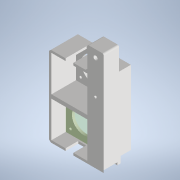
# Autodesk Inventor part: 30_XYTable_Aliexpress_motormount
Saved by Autodesk Inventor 2022 (Build 260153000, 153)
## iProperties
Created: 2021-11-19
Part Number: 30_XYTable_Aliexpress_motormount
Material: Generic
Document SubType Name: Modeling
Designer: diederichbenedict
Density: 1 g/cm^3
Appearance: Default
Author: diederichbenedict
Autodesk Inventor part; units mm, degrees
sketch "Sketch1" plane through (0, 0, 0) normal (0, 0, 1) x (1, 0, 0)
  line L0 (0, 0) -> (-19.7, 0)
  line L1 (-19.7, 0) -> (-19.7, 180)
  line L2 (-19.7, 180) -> (0, 180)
  line L3 (0, 180) -> (0, 38)
  line L4 (0, 38) -> (-19.7, 38)
  dimension "d0" = 19.7
  dimension "d1" = 180
  dimension "d53" = 142
  constraints: 10 end point, 2 parallel, 2 perpendicular, 1 horizontal, 1 point on line
  measures "d0" distance of L1.end L2.end
  measures "d1" distance of L0.end L1.end
  measures "d53" distance between parallel lines of L4 L2
extrude "Extrusion1" add sketch "Sketch1" along normal blind 18
fillet "Fillet1" radius 2 2 edges at (0, 180, 9) (-19.7, 180, 9)
sketch "Sketch2" plane through (0, 0, 0) normal (0, 0, -1) x (-1, 0, 0)
  line L0 (19.7, 178) -> (19.7, 38) projected
  arc A0 (19.7, 178) -> (17.7, 180) centre (17.7, 178) ccw projected
  line L1 (2, 180) -> (17.7, 180) projected
  arc A1 (2, 180) -> (0, 178) centre (2, 178) ccw projected
  line L2 (0, 38) -> (0, 178) projected
  line L3 (-8.568, 22) -> (7.7, 22) construction
  line L4 (-8.568, 12) -> (7.7, 12)
  line L5 (7.7, 32) -> (-8.568, 32)
  arc A2 (-8.568, 32) -> (-8.568, 12) centre (-8.568, 22) ccw
  arc A3 (7.7, 12) -> (7.7, 32) centre (7.7, 22) ccw
  line L6 (19.7, 38) -> (0, 38) projected
  point P0 (0, 0)
  point P1 (-0.434, 22)
  dimension "d5" = 20
  dimension "d6" = 12
  constraints: 8 end point, 4 point on circle, 4 tangent, 2 centre point, 1 horizontal, 1 midpoint, 1 parallel
  measures "d5" diameter of A3
  measures "d6" distance from line of L3.end L0
extrude "Extrusion2" cut sketch "Sketch2" against normal blind 9 contours A2 L5 A3 L4
sketch "Sketch4" plane through (0, 0, 0) normal (0, 0, -1) x (-1, 0, 0)
  line L0 (0, 38) -> (0, 178) projected
  line L1 (19.7, 178) -> (19.7, 38) projected
  arc A0 (19.7, 178) -> (17.7, 180) centre (17.7, 178) ccw projected
  line L2 (2, 180) -> (17.7, 180) projected
  arc A1 (2, 180) -> (0, 178) centre (2, 178) ccw projected
  circle A2 centre (9.7, 52) radius 1.5
  circle A3 centre (9.7, 131) radius 1.5
  line L3 (19.7, 38) -> (0, 38) projected
  point P0 (0, 0)
  dimension "d14" = 3
  dimension "d15" = 3
  dimension "d16" = 10
  dimension "d17" = 10
  dimension "d18" = 49
  dimension "d19" = 79
  constraints: 2 centre point
  measures "d14" diameter of A2
  measures "d15" diameter of A3
  measures "d16" distance from line of A3.centre L1
  measures "d17" distance from line of L1 A2.centre
  measures "d18" distance from line of A3.centre L2
  measures "d19" distance of A2.centre A3.centre
extrude "Extrusion4" cut sketch "Sketch4" against normal blind 110 contours A2 | A3
ref_plane "Work Plane1" through (-61.2, 108.5, -24) normal (0, 0, -1) x (0, 1, 0)
ref_plane "Work Plane3" through (-61.2, 108.5, -11) normal (0, 0, -1) x (0, 1, 0)
sketch "Sketch5" plane through (0, 0, 18) normal (0, 0, 1) x (1, 0, 0)
  circle A0 centre (-9.7, 52) radius 1.5
  circle A1 centre (-9.7, 131) radius 1.5
  line L0 (0, 38) -> (0, 178)
  arc A2 (0, 178) -> (-2, 180) centre (-2, 178) ccw
  line L1 (-2, 180) -> (-17.7, 180)
  arc A3 (-17.7, 180) -> (-19.7, 178) centre (-17.7, 178) ccw
  line L2 (-19.7, 178) -> (-19.7, 38)
  line L3 (-23.7294, 108) -> (-57.6706, 108)
  line L4 (-57.4929, 102.5) -> (-23.9071, 102.5)
  line L5 (-57.6706, 103) -> (-23.7294, 103)
  line L6 (-19.7, 178) -> (-19.7, 38)
  line L7 (-19.7, 108) -> (-61.7, 108)
  line L8 (-61.7, 108) -> (-61.7, 103)
  line L9 (-61.7, 103) -> (-19.7, 103)
  line L10 (-19.7, 103) -> (-19.7, 108)
  line L11 (-61.7, 112.0294) -> (-61.7, 145.9706)
  line L12 (-57.6706, 150) -> (-23.7294, 150)
  line L13 (-23.7294, 61) -> (-57.6706, 61)
  line L14 (0, 38) -> (0, 178)
  line L15 (-19.7, 150) -> (0, 150)
  line L16 (0, 150) -> (0, 61)
  line L17 (0, 61) -> (-19.7, 61)
  line L18 (-19.7, 61) -> (-19.7, 150)
  line L19 (-19.7, 38) -> (0, 38)
  point P0 (0, 0)
  point P1 (0, 110)
  point P2 (-19.7, 2)
  point P3 (0, 32)
  point P4 (-19.7, 103)
  point P5 (-19.7, 103)
extrude "Extrusion5" add sketch "Sketch5" against normal up to surface (29 mm away) contours L17 L2 L15 L0 | L9 L5 L8 L7 L3 L2
sketch "Sketch6" plane through (-19.7, 103, -11) normal (0, 0, -1) x (-1, 0, 0)
  circle A0 centre (-10, 28) radius 1.5 projected
  line L0 (0, -42) -> (-19.7, -42) projected
  line L1 (0, 0) -> (0, -42) projected
  line L2 (42, 0) -> (0, 0) projected
  line L3 (42, 5) -> (42, 0) projected
  line L4 (0, 5) -> (42, 5) projected
  line L5 (0, 47) -> (0, 5) projected
  line L6 (-19.7, 47) -> (0, 47) projected
  line L7 (-19.7, -42) -> (-19.7, 47) projected
  line L8 (0, 5) -> (42, 5) projected
  line L9 (0, 75) -> (0, 47) projected
  line L10 (42, 5) -> (0, 5)
  line L11 (0, 5) -> (0, 47)
  line L12 (0, 47) -> (42, 47)
  line L13 (42, 47) -> (42, 5)
  circle A1 centre (36.5, 10.5) radius 1.5 projected
  circle A2 centre (5.5, 10.5) radius 1.5 projected
  circle A3 centre (5.5, 41.5) radius 1.5 projected
  circle A4 centre (36.5, 41.5) radius 1.5 projected
  circle A5 centre (21, 26) radius 15 projected
  point P0 (-19.7, -103)
  constraints: 8 end point, 2 parallel, 1 horizontal, 1 perpendicular
extrude "Extrusion6" add sketch "Sketch6" along normal blind 3
ref_plane "Work Plane2" through (-40.7, 82, 1) normal (0, 0, -1) x (1, 0, 0)
sketch "Sketch7" plane through (-40.7, 82, 1) normal (0, 0, -1) x (1, 0, 0)
  line L0 (-21, -68) -> (40.7, -68) projected
  line L1 (40.7, -68) -> (40.7, 21) projected
  line L2 (40.7, 21) -> (21, 21) projected
  line L3 (21, 21) -> (21, -21) projected
  line L4 (21, -21) -> (-21, -21) projected
  line L5 (-21, -21) -> (-21, -68) projected
  circle A0 centre (31, -49) radius 1.5 projected
  circle A1 centre (0, -47) radius 15 projected
  circle A2 centre (-15.5, -62.5) radius 1.5 projected
  circle A3 centre (15.5, -62.5) radius 1.5 projected
  circle A4 centre (15.5, -31.5) radius 1.5 projected
  circle A5 centre (-15.5, -31.5) radius 1.5 projected
  line L6 (21, 21) -> (40.7, 21) projected
  line L7 (21, -21) -> (-21, -21) projected
  line L8 (21, 21) -> (-21, 21)
  line L9 (-21, 21) -> (-21, -21)
  line L10 (-21, -21) -> (21, -21)
  line L11 (21, -21) -> (21, 21)
  circle A6 centre (-15.5, 15.5) radius 1.5 projected
  circle A7 centre (-15.5, -15.5) radius 1.5 projected
  circle A8 centre (15.5, -15.5) radius 1.5 projected
  circle A9 centre (15.5, 15.5) radius 1.5 projected
  circle A10 centre (0, 0) radius 14 projected
  point P0 (40.7, 82)
  point P1 (34.7, 21)
  constraints: 8 end point, 2 parallel, 1 horizontal, 1 perpendicular
extrude "Extrusion7" add sketch "Sketch7" along normal blind 3 contours L9 L8 L3 L4
sketch "Sketch8" plane through (-61.7, 103, 18) normal (-1, 0, 0) x (0, 0, 1)
  line L0 (0, 0) -> (-17, 0) projected
  line L1 (0, 5) -> (0, 0) projected
  line L2 (0, 5) -> (-29, 5) projected
  line L3 (-29, 5) -> (-29, 47) projected
  line L4 (-29, 47) -> (-32, 47) projected
  line L5 (-32, 0) -> (-32, 47) projected
  line L6 (-20, 0) -> (-32, 0) projected
  line L7 (-20, -42) -> (-20, 0) projected
  line L8 (-17, -42) -> (-20, -42) projected
  line L9 (-17, -42) -> (-17, 0) projected
  line L10 (-32, 47) -> (-32, -42) projected
  line L11 (-32, 47) -> (0, 47)
  line L12 (0, 47) -> (0, 0)
  line L13 (0, 0) -> (-32, 0)
  line L14 (-32, 0) -> (-32, 47)
  line L15 (0, 0) -> (-20, 0)
  line L16 (-20, 0) -> (-20, -42)
  line L17 (-20, -42) -> (0, -42)
  line L18 (0, -42) -> (0, 0)
  point P0 (-18, -103)
  point P1 (-23, 7)
  constraints: 16 end point, 4 parallel, 2 horizontal, 2 perpendicular, 2 other
extrude "Extrusion8" add sketch "Sketch8" along normal blind 3
sketch "Sketch9" plane through (-19.7, 150, 0) normal (0, 1, 0) x (1, 0, 0)
  line L0 (19.7, 0) -> (0, 0) projected
  line L1 (19.7, 0) -> (19.7, 14) projected
  line L2 (19.7, 14) -> (-45, 14) projected
  line L3 (-45, -18) -> (-45, 14) projected
  line L4 (-42, -18) -> (-45, -18) projected
  line L5 (-42, -18) -> (-42, 11) projected
  line L6 (-42, 11) -> (0, 11) projected
  line L7 (0, 0) -> (0, 11) projected
  line L8 (-42, -18) -> (0, -18) projected
  line L9 (-42, 11) -> (0, 11) projected
  line L10 (-42, -18) -> (0, -18)
  line L11 (0, -18) -> (0, 11)
  line L12 (0, 11) -> (-42, 11)
  line L13 (-42, 11) -> (-42, -18)
  constraints: 8 end point, 2 parallel, 1 horizontal, 1 perpendicular
extrude "Extrusion9" add sketch "Sketch9" along normal blind 3
sketch "Sketch10" plane through (-19.7, 61, 0) normal (0, -1, 0) x (1, 0, 0)
  line L0 (0, 0) -> (19.7, 0) projected
  line L1 (0, 1) -> (0, 0) projected
  line L2 (0, 1) -> (-42, 1) projected
  line L3 (-42, 1) -> (-42, 18) projected
  line L4 (-42, 18) -> (-45, 18) projected
  line L5 (-45, -2) -> (-45, 18) projected
  line L6 (0, -2) -> (-45, -2) projected
  line L7 (0, -2) -> (0, -14) projected
  line L8 (19.7, -14) -> (0, -14) projected
  line L9 (-42, 1) -> (0, 1) projected
  line L10 (0, -11) -> (0, 18) projected
  line L11 (-42, 1) -> (0, 1)
  line L12 (0, 1) -> (0, 18)
  line L13 (0, 18) -> (-42, 18)
  line L14 (-42, 18) -> (-42, 1)
  line L15 (19.7, 0) -> (19.7, -14) projected
  point P0 (19.7, 0)
  constraints: 8 end point, 2 parallel, 1 horizontal, 1 perpendicular
extrude "Extrusion10" add sketch "Sketch10" along normal blind 3
sketch "Sketch11" plane through (0, 0, 18) normal (0, 0, 1) x (1, 0, 0)
  line L0 (-61.7, 61) -> (-61.7, 103) projected
  line L1 (-61.7, 103) -> (-19.7, 103) projected
  line L2 (-19.7, 103) -> (-19.7, 61) projected
  line L3 (-19.7, 61) -> (-61.7, 61) projected
  line L4 (-19.7, 150) -> (-19.7, 108) projected
  line L5 (-19.7, 108) -> (-61.7, 108) projected
  line L6 (-61.7, 108) -> (-61.7, 150) projected
  line L7 (-61.7, 150) -> (-19.7, 150) projected
  circle A0 centre (-9.7, 52) radius 1.5 projected
  circle A1 centre (-9.7, 131) radius 1.5 projected
  line L8 (-64.7, 153) -> (-64.7, 58) projected
  line L9 (-19.7, 58) -> (-64.7, 58) projected
  line L10 (-19.7, 58) -> (-19.7, 38) projected
  line L11 (0, 38) -> (0, 178) projected
  arc A2 (0, 178) -> (-2, 180) centre (-2, 178) ccw projected
  line L12 (-2, 180) -> (-17.7, 180) projected
  arc A3 (-17.7, 180) -> (-19.7, 178) centre (-17.7, 178) ccw projected
  line L13 (-19.7, 178) -> (-19.7, 153) projected
  line L14 (-64.7, 153) -> (-19.7, 153) projected
  line L15 (-61.95, 103.25) -> (-61.95, 60.75)
  line L16 (-61.95, 60.75) -> (-19.45, 60.75)
  line L17 (-19.45, 60.75) -> (-19.45, 103.25)
  line L18 (-19.45, 103.25) -> (-61.95, 103.25)
  line L19 (-61.95, 150.25) -> (-61.95, 107.75)
  line L20 (-61.95, 107.75) -> (-19.45, 107.75)
  line L21 (-19.45, 107.75) -> (-19.45, 150.25)
  line L22 (-19.45, 150.25) -> (-61.95, 150.25)
  line L23 (-19.7, 38) -> (0, 38) projected
  point P0 (0, 0)
  dimension "d35" = 0.25
  dimension "d36" = 0.25
  constraints: 16 end point, 6 other
  measures "d35" distance between parallel lines of L0 L15
  measures "d36" distance between parallel lines of L6 L19
extrude "Extrusion11" cut sketch "Sketch11" against normal up to surface (17 mm away) contours L0 L1 L2 L3 | L4 L5 L6 L7 | L18 L17 L16 L15 | L22 L21 L20 L19
sketch "Sketch12" plane through (0, 0, 18) normal (0, 0, 1) x (1, 0, 0)
  line L0 (-61.95, 107.75) -> (-61.95, 150.25) projected
  line L1 (-61.95, 150.25) -> (-19.45, 150.25) projected
  line L2 (-19.45, 150.25) -> (-19.45, 107.75) projected
  line L3 (-19.45, 107.75) -> (-61.95, 107.75) projected
  line L4 (-61.95, 103.25) -> (-19.45, 103.25) projected
  line L5 (-19.45, 103.25) -> (-19.45, 60.75) projected
  line L6 (-19.45, 60.75) -> (-61.95, 60.75) projected
  line L7 (-61.95, 60.75) -> (-61.95, 103.25) projected
  circle A0 centre (-9.7, 52) radius 1.5 projected
  circle A1 centre (-9.7, 131) radius 1.5 projected
  line L8 (-64.7, 153) -> (-64.7, 58) projected
  line L9 (-19.7, 58) -> (-64.7, 58) projected
  line L10 (-19.7, 58) -> (-19.7, 38) projected
  line L11 (0, 38) -> (0, 178) projected
  arc A2 (0, 178) -> (-2, 180) centre (-2, 178) ccw projected
  line L12 (-2, 180) -> (-17.7, 180) projected
  arc A3 (-17.7, 180) -> (-19.7, 178) centre (-17.7, 178) ccw projected
  line L13 (-19.7, 178) -> (-19.7, 153) projected
  line L14 (-64.7, 153) -> (-19.7, 153) projected
  line L15 (-19.7, 38) -> (0, 38) projected
  point P0 (0, 0)
ref_plane "Work Plane4" through (-61.2, 108.5, -11) normal (0, 0, -1) x (0, 1, 0)
extrude "Extrusion12" cut sketch "Sketch12" against normal up to surface (29 mm away) contours L0 L1 L2 L3
chamfer "Chamfer1" distance 2 angle 45 6 edges at (-64.7, 58, 8) (-64.7, 153, 2) (-64.7, 103, -8) (-19.7, 58, 9) (-19.7, 58, -8) (-19.7, 153, 9)
sketch "Sketch13" plane through (-19.7, 103, -14) normal (0, 0, -1) x (-1, 0, 0)
  circle A0 centre (-10, 28) radius 1.5 projected
  circle A1 centre (-10, -51) radius 1.5 projected
  point P0 (-19.7, -103)
hole "Hole1" at (-9.7, 52, -14) at (-9.7, 131, -14) direction (0, 0, 1) diameter 2.5 end through all counterbore diameter 5 counterbore depth 20
sketch "Sketch14" plane through (-19.7, 103, -14) normal (0, 0, -1) x (-1, 0, 0)
  circle A0 centre (-10, 28) radius 2.5 projected
  circle A1 centre (36.5, 10.5) radius 1.5 projected
  circle A2 centre (5.5, 10.5) radius 1.5 projected
  circle A3 centre (5.5, 41.5) radius 1.5 projected
  circle A4 centre (36.5, 41.5) radius 1.5 projected
  circle A5 centre (21, 26) radius 15 projected
  line L0 (0, -43) -> (-2, -45) projected
  line L1 (0, 0) -> (0, -43) projected
  line L2 (0, 0) -> (43, 0) projected
  line L3 (45, 2) -> (43, 0) projected
  line L4 (45, 2) -> (45, 48) projected
  line L5 (43, 50) -> (45, 48) projected
  line L6 (-19.7, 50) -> (43, 50) projected
  line L7 (-19.7, -45) -> (-19.7, 50) projected
  line L8 (-2, -45) -> (-19.7, -45) projected
  circle A6 centre (21, -21) radius 3.5 projected
  line L9 (-32.7587, -50.6684) -> (7.6884, -72.8519)
  line L10 (7.6884, -72.8519) -> (27.6493, -33.2508)
  circle A7 centre (21, -21) radius 14 projected
  line L11 (27.6013, -33.346) -> (5.5, -11.6661)
  line L12 (5.5, -11.6661) -> (-32.7587, -50.6684)
  point P0 (-19.7, -103)
  point P1 (18.9527, -18.1612)
  constraints: 8 end point, 1 perpendicular, 1 point on line, 4 other
extrude "Extrusion13" cut sketch "Sketch14" against normal up to surface (12 mm away) contours L1 L12 L11 A7 L10 L9 L7 L8 L0 | L0 L8 L7 L12 L1 | L11 A7 | A6 picked at (13.3334, -27.485)
sketch "Sketch15" plane through (0, 0, -14) normal (0, 0, -1) x (-1, 0, 0)
  circle A0 centre (9.7, 52) radius 2.5 projected
  circle A1 centre (9.5, 171.1) radius 2.5
  line L0 (2, 180) -> (17.7, 180) projected
  line L1 (0, 153) -> (0, 178) projected
  circle A2 centre (9.85, 121.1) radius 2.9049
  circle A3 centre (9.5, 61.1) radius 2.7549
  point P0 (0, 0)
  dimension "d54" = 5
  dimension "d55" = 8.9
  dimension "d70" = 9.5
  dimension "d71" = 50
  dimension "d72" = 60
  constraints: 3 centre point
  measures "d54" diameter of A1
  measures "d55" distance from line of A1.centre L0
  measures "d70" distance from line of A1.centre L1
  measures "d71" vertical distance of A2.centre A1.centre
  measures "d72" vertical distance of A3.centre A2.centre
sketch "Skizze16" plane through (0, 0, 18) normal (0, 0, 1) x (1, 0, 0)
  line L0 (-64.7, 151) -> (-62.7, 153) projected
  line L1 (-64.7, 151) -> (-64.7, 60) projected
  line L2 (-62.7, 58) -> (-64.7, 60) projected
  line L3 (-21.7, 58) -> (-62.7, 58) projected
  line L4 (-19.7, 56) -> (-21.7, 58) projected
  line L5 (-19.7, 56) -> (-19.7, 38) projected
  line L6 (-19.7, 38) -> (0, 38) projected
  line L7 (0, 38) -> (0, 178) projected
  arc A0 (0, 178) -> (-2, 180) centre (-2, 178) ccw projected
  line L8 (-2, 180) -> (-17.7, 180) projected
  arc A1 (-17.7, 180) -> (-19.7, 178) centre (-17.7, 178) ccw projected
  line L9 (-19.7, 178) -> (-19.7, 155) projected
  line L10 (-21.7, 153) -> (-19.7, 155) projected
  line L11 (-62.7, 153) -> (-21.7, 153) projected
  line L12 (-61.95, 107.75) -> (-61.95, 150.25) projected
  line L13 (-61.95, 150.25) -> (-19.45, 150.25) projected
  line L14 (-19.45, 150.25) -> (-19.45, 107.75) projected
  line L15 (-19.45, 107.75) -> (-61.95, 107.75) projected
  line L16 (-61.95, 103.25) -> (-19.45, 103.25) projected
  line L17 (-19.45, 103.25) -> (-19.45, 60.75) projected
  line L18 (-19.45, 60.75) -> (-61.95, 60.75) projected
  line L19 (-61.95, 60.75) -> (-61.95, 103.25) projected
  circle A2 centre (-9.7, 52) radius 1.5 projected
  circle A3 centre (-9.7, 131) radius 1.5 projected
  line L20 (-45.3346, 64) -> (-36.0654, 64)
  line L21 (-36.0654, 64) -> (-36.0654, 56)
  line L22 (-36.0654, 56) -> (-45.3346, 56)
  line L23 (-45.3346, 56) -> (-45.3346, 64)
  line L24 (-45.3346, 64) -> (-36.0654, 56) construction
  line L25 (-36.0654, 64) -> (-45.3346, 56) construction
  point P0 (0, 0)
  point P1 (-40.7, 60)
  constraints: 12 end point, 2 midpoint, 2 parallel, 1 horizontal, 1 perpendicular
extrude "Extrusion15" cut sketch "Skizze16" against normal blind 15 contours L23 L18 L21 L3 | L3 L21 L22 L23 | L23 L20 L21 L18
sketch "Skizze17" plane through (0, 0, 18) normal (0, 0, 1) x (1, 0, 0)
  line L0 (-36.0654, 60.75) -> (-36.0654, 58) projected
  line L1 (-21.7, 58) -> (-36.0654, 58) projected
  line L2 (-19.7, 56) -> (-21.7, 58) projected
  line L3 (-19.7, 56) -> (-19.7, 38) projected
  line L4 (-19.7, 38) -> (0, 38) projected
  line L5 (0, 38) -> (0, 178) projected
  arc A0 (0, 178) -> (-2, 180) centre (-2, 178) ccw projected
  line L6 (-2, 180) -> (-17.7, 180) projected
  arc A1 (-17.7, 180) -> (-19.7, 178) centre (-17.7, 178) ccw projected
  line L7 (-19.7, 178) -> (-19.7, 155) projected
  line L8 (-21.7, 153) -> (-19.7, 155) projected
  line L9 (-62.7, 153) -> (-21.7, 153) projected
  line L10 (-64.7, 151) -> (-62.7, 153) projected
  line L11 (-64.7, 151) -> (-64.7, 60) projected
  line L12 (-62.7, 58) -> (-64.7, 60) projected
  line L13 (-45.3346, 58) -> (-62.7, 58) projected
  line L14 (-45.3346, 58) -> (-45.3346, 60.75) projected
  line L15 (-45.3346, 60.75) -> (-61.95, 60.75) projected
  line L16 (-61.95, 60.75) -> (-61.95, 103.25) projected
  line L17 (-61.95, 103.25) -> (-19.45, 103.25) projected
  line L18 (-19.45, 103.25) -> (-19.45, 60.75) projected
  line L19 (-19.45, 60.75) -> (-36.0654, 60.75) projected
  line L20 (-61.95, 107.75) -> (-61.95, 150.25) projected
  line L21 (-61.95, 150.25) -> (-19.45, 150.25) projected
  line L22 (-19.45, 150.25) -> (-19.45, 107.75) projected
  line L23 (-19.45, 107.75) -> (-61.95, 107.75) projected
  circle A2 centre (-9.7, 52) radius 1.5 projected
  circle A3 centre (-9.7, 131) radius 1.5 projected
  line L24 (-61.95, 150.25) -> (-19.45, 150.25) projected
  line L25 (-45.3346, 150.25) -> (-36.0654, 150.25)
  line L26 (-36.0654, 150.25) -> (-36.0654, 153)
  line L27 (-36.0654, 153) -> (-45.3346, 153)
  line L28 (-45.3346, 153) -> (-45.3346, 150.25)
  point P0 (0, 0)
  constraints: 8 end point, 2 parallel, 2 point on line, 1 horizontal, 1 perpendicular
extrude "Extrusion16" cut sketch "Skizze17" against normal blind 25 contours L9 L26 L21 L28
sketch "Skizze18" plane through (-40.7, 82, -2) normal (0, 0, -1) x (-1, 0, 0)
  circle A0 centre (-31, -30) radius 2.5 projected
  line L0 (-19, -24) -> (-40.7, -24) projected
  line L1 (-40.7, -44) -> (-40.7, -24) projected
  line L2 (-21, -44) -> (-40.7, -44) projected
  line L3 (-21, -26) -> (-21, -44) projected
  line L4 (-19, -24) -> (-21, -26) projected
  line L5 (-10.4215, -54.1339) -> (-43.6048, -54.1339)
  line L6 (-43.6048, -54.1339) -> (-43.6048, -24)
  line L7 (-43.6048, -24) -> (-10.4215, -24)
  line L8 (-10.4215, -24) -> (-10.4215, -54.1339)
  point P0 (-40.7, -82)
  constraints: 8 end point, 2 parallel, 1 horizontal, 1 perpendicular
extrude "Extrusion17" cut sketch "Skizze18" against normal through all contours A0 | L4 L3 L2 L1 L0 | L7 L8 L5 L6 L1 L2 L3 L4
sketch "Skizze19" plane through (-19.7, 58, 0) normal (0, -1, 0) x (1, 0, 0)
  line L0 (19.7, 18) -> (-16.3654, 18) projected
  line L1 (-16.3654, 18) -> (-16.3654, 3) projected
  line L2 (-16.3654, 3) -> (-25.6346, 3) projected
  line L3 (-25.6346, 3) -> (-25.6346, 18) projected
  line L4 (-25.6346, 18) -> (-43, 18) projected
  line L5 (-43, -2) -> (-43, 18) projected
  line L6 (-43, -2) -> (19.7, -2) projected
  line L7 (19.7, -2) -> (19.7, 18) projected
  line L8 (19.7, 18) -> (12.7, 18)
  line L9 (12.7, 18) -> (12.7, 11)
  line L10 (12.7, 11) -> (19.7, 11)
  line L11 (19.7, 11) -> (19.7, 18)
  point P0 (19.7, 0)
  dimension "d66" = 7
  dimension "d67" = 7
  constraints: 8 end point, 2 parallel, 1 horizontal, 1 perpendicular
  measures "d66" distance of L10.end L9.end
  measures "d67" distance of L9.end L8.end
extrude "Extrusion18" cut sketch "Skizze19" against normal blind 100 contours L7 L10 L9 L0
hole "Bohrung2" at (-9.5, 171.1, -14) at (-9.85, 121.1, -14) at (-9.5, 61.1, -14) direction (0, 0, 1) diameter 4.5 end through all counterbore diameter 9 counterbore depth 15
body "Solid1"
